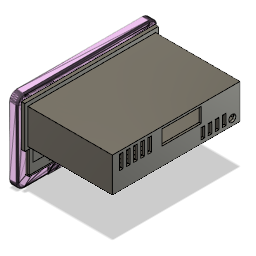
Headunit (Autodesk Fusion 360 design; units mm, degrees)
Autodesk Fusion 360 part; units mm, degrees
sketch "Sketch1" plane through (0, 0, 0) normal (0, 1, 0) x (1, 0, 0)
  line L0 (50, 100) -> (50, -80)
  line L1 (50, -80) -> (1, -80)
  line L2 (1, -80) -> (1, 100)
  line L3 (1, 100) -> (50, 100)
  constraint vertical L0
  constraint perpendicular L0 L1
  constraint perpendicular L1 L2
  constraint perpendicular L0 L3
extrude "Extrude1" add sketch "Sketch1" along normal blind 120 makes body 1
move_body "Move1" bodies 1 to x (0, 1, 0) y (-1, 0, 0) z (0, 0, 1) at (1, -1, 0)
shell "Shell1" thickness 3 removed faces 1 at (-119, 16.3333, -40) on bodies 1
hole "Hole1" at (1, 9.462, -88.8888) direction (-1, 0, 0) diameter 10 depth 60 tip angle 118 bodies 1
sketch "Sketch2" plane through (1, 0, 0) normal (1, 0, 0) x (0, 0, -1)
  circle A0 centre (88.8888, 9.462) radius 5
  line L0 (-80, 0) -> (100, 0)
  line L1 (100, 0) -> (100, 49)
  line L2 (100, 49) -> (-80, 49)
  line L3 (-80, 49) -> (-80, 0)
  line L4 (-60, 40) -> (-55.5469, 40)
  line L5 (-55.5469, 40) -> (-55.5469, 10)
  line L6 (-55.5469, 10) -> (-60, 10)
  line L7 (-60, 10) -> (-60, 40)
  constraint perpendicular L3 L4
  constraint perpendicular L4 L5
  constraint perpendicular L5 L6
  constraint perpendicular L4 L7
extrude "Extrude2" add sketch "Sketch2" along normal blind 40 contours L4 L5 L6 L7 bodies 1
delete_face "DeleteFace1" 1 faces at (14.3333, 20, 60) on bodies 1
sketch "Sketch5" plane through (1, 0, 0) normal (1, 0, 0) x (0, 0, -1)
  circle A0 centre (88.8888, 9.462) radius 5
  line L0 (-80, 49) -> (-80, 0)
  line L1 (-80, 0) -> (100, 0)
  line L2 (100, 0) -> (100, 49)
  line L3 (100, 49) -> (-80, 49)
  line L4 (-70, 40) -> (-64.9792, 40)
  line L5 (-64.9792, 40) -> (-64.9792, 10)
  line L6 (-64.9792, 10) -> (-67.4896, 10)
  line L7 (-67.4896, 10) -> (-70, 10)
  line L8 (-70, 10) -> (-70, 40)
  line L9 (-60, 40) -> (-54.6378, 40)
  line L10 (-54.6378, 40) -> (-54.6378, 10)
  line L11 (-54.6378, 10) -> (-60, 10)
  line L12 (-60, 10) -> (-60, 40)
  line L13 (-50, 40) -> (-44.6795, 40)
  line L14 (-44.6795, 40) -> (-44.6795, 10)
  line L15 (-44.6795, 10) -> (-47.3397, 10)
  line L16 (-47.3397, 10) -> (-50, 10)
  line L17 (-50, 10) -> (-50, 40)
  line L18 (-40, 40) -> (-34.7211, 40)
  line L19 (-34.7211, 40) -> (-34.7211, 10)
  line L20 (-34.7211, 10) -> (-40, 10)
  line L21 (-40, 10) -> (-40, 40)
  line L22 (-30, 40) -> (-24.7628, 40)
  line L23 (-24.7628, 40) -> (-24.7628, 10)
  line L24 (-24.7628, 10) -> (-30, 10)
  line L25 (-30, 10) -> (-30, 40)
  line L26 (-20, 40) -> (-14.8044, 40)
  line L27 (-14.8044, 40) -> (-14.8044, 10)
  line L28 (-14.8044, 10) -> (-20, 10)
  line L29 (-20, 10) -> (-20, 40)
  constraint parallel L3 L4
  constraint perpendicular L4 L5
  constraint perpendicular L5 L6
  constraint perpendicular L4 L8
  constraint perpendicular L5 L9
  constraint perpendicular L9 L10
  constraint perpendicular L10 L11
  constraint perpendicular L9 L12
  constraint perpendicular L10 L13
  constraint perpendicular L13 L14
  constraint perpendicular L14 L15
  constraint perpendicular L14 L16
  constraint perpendicular L13 L17
  constraint perpendicular L14 L18
  constraint perpendicular L18 L19
  constraint perpendicular L19 L20
  constraint perpendicular L18 L21
  constraint perpendicular L19 L22
  constraint perpendicular L22 L23
  constraint perpendicular L19 L24
  constraint perpendicular L22 L25
  constraint perpendicular L23 L26
  constraint perpendicular L26 L27
  constraint perpendicular L27 L28
  constraint perpendicular L26 L29
extrude "Extrude4" cut sketch "Sketch5" against normal blind 30 contours L4 L5 L6 L7 L8 | L9 L10 L11 L12 | L13 L14 L15 L16 L17 | L18 L19 L20 L21 | L22 L23 L24 L25 | L26 L27 L28 L29 bodies 1
sketch "Sketch6" plane through (-119, 0, 0) normal (-1, 0, 0) x (0, 0, 1)
  line L0 (-97, 3) -> (-97, 46)
  line L1 (-97, 46) -> (77, 46)
  line L2 (77, 46) -> (77, 3)
  line L3 (77, 3) -> (-97, 3)
  line L4 (-100, 0) -> (80, 0)
  line L5 (80, 0) -> (80, 49)
  line L6 (80, 49) -> (-100, 49)
  line L7 (-100, 49) -> (-100, 0)
  line L8 (-104.1759, 54.472) -> (84.2667, 54.472)
  line L9 (84.2667, 54.472) -> (84.2667, -4.1291)
  line L10 (84.2667, -4.1291) -> (-103.7929, -4.1291)
  line L11 (-103.7929, -4.1291) -> (-104.1759, 54.472)
  constraint parallel L6 L8
  constraint perpendicular L8 L9
  constraint perpendicular L9 L10
extrude "Extrude5" add sketch "Sketch6" along normal blind 5 separate body contours L8 L9 L10 L11 makes body 2
move_body "Move4" bodies 2 to x (1, 0, 0) y (0, 1, 0) z (0, 0, 1) at (1, 0, 0)
mesh "Mesh1" [no effect]
sketch "Sketch7" plane through (-2, 0, 0) normal (-1, 0, 0) x (0, 0, 1)
  line L0 (44.6795, 10) -> (44.6795, 40)
  line L1 (44.6795, 40) -> (50, 40)
  line L2 (50, 40) -> (50, 10)
  line L3 (50, 10) -> (44.6795, 10)
  line L4 (14.8044, 10) -> (14.8044, 40)
  line L5 (14.8044, 40) -> (20, 40)
  line L6 (20, 40) -> (20, 10)
  line L7 (20, 10) -> (14.8044, 10)
  line L8 (54.6378, 10) -> (54.6378, 40)
  line L9 (54.6378, 40) -> (60, 40)
  line L10 (60, 40) -> (60, 10)
  line L11 (60, 10) -> (54.6378, 10)
  line L12 (34.7211, 10) -> (34.7211, 40)
  line L13 (34.7211, 40) -> (40, 40)
  line L14 (40, 40) -> (40, 10)
  line L15 (40, 10) -> (34.7211, 10)
  line L16 (24.7628, 10) -> (24.7628, 40)
  line L17 (24.7628, 40) -> (30, 40)
  line L18 (30, 40) -> (30, 10)
  line L19 (30, 10) -> (24.7628, 10)
  line L20 (64.9792, 10) -> (64.9792, 40)
  line L21 (64.9792, 40) -> (70, 40)
  line L22 (70, 40) -> (70, 10)
  line L23 (70, 10) -> (64.9792, 10)
  circle A0 centre (-88.8888, 9.462) radius 5
  line L24 (-97, 3) -> (77, 3)
  line L25 (77, 3) -> (77, 46)
  line L26 (77, 46) -> (-97, 46)
  line L27 (-97, 46) -> (-97, 3)
  line L28 (-97, 24.9908) -> (-92, 24.9908)
  line L29 (-92, 24.9908) -> (-92, 28)
  line L30 (-97, 28) -> (-97, 24.9908)
  line L31 (-97, 24.9908) -> (-97, 23.492)
  line L32 (-97, 24.9908) -> (-97, 22.5)
  line L33 (-92, 22.5) -> (-97, 22.5)
  line L34 (-92, 22.5) -> (-92, 20.5)
  line L35 (-92, 20.5) -> (-91.9643, 13.4043)
  line L36 (-91.9643, 13.4043) -> (-97, 13.4)
  line L37 (-97, 22.5) -> (-97, 13.4)
  line L38 (-92, 28) -> (-92, 46)
  line L39 (-97, 46) -> (-97, 24.9908)
  constraint coincident L27 L28.start
  constraint perpendicular L27 L28
  constraint perpendicular L28 L29
  constraint coincident L27 L30.start
  constraint coincident L27 L31.end
  constraint coincident L27 L32.end
  constraint perpendicular L27 L33
  constraint coincident A0 L35.end
  constraint coincident L27 L36.end
  constraint coincident L26 L38.end
  constraint coincident L26.end L27.start
extrude "Extrude6" add sketch "Sketch7" along normal blind 100 contours L27 L33 L34 L35 L36 L37 | L26 L27 L28 L29 L30 L38 L39 bodies 1
sketch "Sketch8" plane through (-2, 0, 0) normal (-1, 0, 0) x (0, 0, 1)
  line L0 (-91.9643, 13.4043) -> (-97, 13.4)
  line L1 (-97, 13.4) -> (-97, 3)
  line L2 (-97, 3) -> (77, 3)
  line L3 (77, 3) -> (77, 46)
  line L4 (77, 46) -> (-92, 46)
  line L5 (-92, 46) -> (-92, 24.9908)
  line L6 (-92, 24.9908) -> (-97, 24.9908)
  line L7 (-97, 24.9908) -> (-97, 22.5)
  line L8 (-97, 22.5) -> (-92, 22.5)
  line L9 (-92, 22.5) -> (-92, 20.5)
  line L10 (-92, 20.5) -> (-91.9643, 13.4043)
  circle A0 centre (-88.8888, 9.462) radius 5
  line L11 (64.9792, 10) -> (64.9792, 40)
  line L12 (64.9792, 40) -> (70, 40)
  line L13 (70, 40) -> (70, 10)
  line L14 (70, 10) -> (64.9792, 10)
  line L15 (24.7628, 10) -> (24.7628, 40)
  line L16 (24.7628, 40) -> (30, 40)
  line L17 (30, 40) -> (30, 10)
  line L18 (30, 10) -> (24.7628, 10)
  line L19 (34.7211, 10) -> (34.7211, 40)
  line L20 (34.7211, 40) -> (40, 40)
  line L21 (40, 40) -> (40, 10)
  line L22 (40, 10) -> (34.7211, 10)
  line L23 (54.6378, 10) -> (54.6378, 40)
  line L24 (54.6378, 40) -> (60, 40)
  line L25 (60, 40) -> (60, 10)
  line L26 (60, 10) -> (54.6378, 10)
  line L27 (14.8044, 10) -> (14.8044, 40)
  line L28 (14.8044, 40) -> (20, 40)
  line L29 (20, 40) -> (20, 10)
  line L30 (20, 10) -> (14.8044, 10)
  line L31 (44.6795, 10) -> (44.6795, 40)
  line L32 (44.6795, 40) -> (50, 40)
  line L33 (50, 40) -> (50, 10)
  line L34 (50, 10) -> (44.6795, 10)
  line L35 (77, 25.0463) -> (71.9692, 24.9908)
  line L36 (71.9692, 24.9908) -> (71.9692, 46)
  line L37 (77, 22.1504) -> (72, 22.1504)
  line L38 (72, 22.1504) -> (72, 3)
  constraint coincident L3 L35.start
  constraint coincident L4 L36.end
  constraint perpendicular L4 L36
  constraint coincident L3 L37.start
  constraint perpendicular L3 L37
  constraint coincident L2 L38.end
extrude "Extrude7" add sketch "Sketch8" along normal blind 100 contours L3 L4 L35 L36 bodies 1
sketch "Sketch9" plane through (-2, 0, 0) normal (-1, 0, 0) x (0, 0, 1)
  line L0 (71.9692, 24.9908) -> (71.9692, 46)
  line L1 (71.9692, 46) -> (-92, 46)
  line L2 (-92, 46) -> (-92, 24.9908)
  line L3 (-92, 24.9908) -> (-97, 24.9908)
  line L4 (-97, 24.9908) -> (-97, 22.5)
  line L5 (-97, 22.5) -> (-92, 22.5)
  line L6 (-92, 22.5) -> (-92, 20.5)
  line L7 (-92, 20.5) -> (-91.9643, 13.4043)
  circle A0 centre (-88.8888, 9.462) radius 5
  line L8 (-91.9643, 13.4043) -> (-97, 13.4)
  line L9 (-97, 13.4) -> (-97, 3)
  line L10 (-97, 3) -> (77, 3)
  line L11 (77, 3) -> (77, 25.0463)
  line L12 (77, 25.0463) -> (71.9692, 24.9908)
  line L13 (64.9792, 10) -> (64.9792, 40)
  line L14 (64.9792, 40) -> (70, 40)
  line L15 (70, 40) -> (70, 10)
  line L16 (70, 10) -> (64.9792, 10)
  line L17 (24.7628, 10) -> (24.7628, 40)
  line L18 (24.7628, 40) -> (30, 40)
  line L19 (30, 40) -> (30, 10)
  line L20 (30, 10) -> (24.7628, 10)
  line L21 (34.7211, 10) -> (34.7211, 40)
  line L22 (34.7211, 40) -> (40, 40)
  line L23 (40, 40) -> (40, 10)
  line L24 (40, 10) -> (34.7211, 10)
  line L25 (54.6378, 10) -> (54.6378, 40)
  line L26 (54.6378, 40) -> (60, 40)
  line L27 (60, 40) -> (60, 10)
  line L28 (60, 10) -> (54.6378, 10)
  line L29 (14.8044, 10) -> (14.8044, 40)
  line L30 (14.8044, 40) -> (20, 40)
  line L31 (20, 40) -> (20, 10)
  line L32 (20, 10) -> (14.8044, 10)
  line L33 (44.6795, 10) -> (44.6795, 40)
  line L34 (44.6795, 40) -> (50, 40)
  line L35 (50, 40) -> (50, 10)
  line L36 (50, 10) -> (44.6795, 10)
  line L37 (77, 22.5204) -> (72, 22.5204)
  line L38 (72, 22.5204) -> (72, 3)
  constraint coincident L11 L37.start
  constraint perpendicular L11 L37
  constraint coincident L10 L38.end
extrude "Extrude8" add sketch "Sketch9" along normal blind 100 contours L10 L11 L37 L38 bodies 1
sketch "Sketch10" plane through (-2, 0, 0) normal (-1, 0, 0) x (0, 0, 1)
  line L0 (44.6795, 10) -> (44.6795, 40)
  line L1 (44.6795, 40) -> (50, 40)
  line L2 (50, 40) -> (50, 10)
  line L3 (50, 10) -> (44.6795, 10)
  line L4 (14.8044, 10) -> (14.8044, 40)
  line L5 (14.8044, 40) -> (20, 40)
  line L6 (20, 40) -> (20, 10)
  line L7 (20, 10) -> (14.8044, 10)
  line L8 (54.6378, 10) -> (54.6378, 40)
  line L9 (54.6378, 40) -> (60, 40)
  line L10 (60, 40) -> (60, 10)
  line L11 (60, 10) -> (54.6378, 10)
  line L12 (34.7211, 10) -> (34.7211, 40)
  line L13 (34.7211, 40) -> (40, 40)
  line L14 (40, 40) -> (40, 10)
  line L15 (40, 10) -> (34.7211, 10)
  line L16 (24.7628, 10) -> (24.7628, 40)
  line L17 (24.7628, 40) -> (30, 40)
  line L18 (30, 40) -> (30, 10)
  line L19 (30, 10) -> (24.7628, 10)
  line L20 (64.9792, 10) -> (64.9792, 40)
  line L21 (64.9792, 40) -> (70, 40)
  line L22 (70, 40) -> (70, 10)
  line L23 (70, 10) -> (64.9792, 10)
  line L24 (72, 3) -> (72, 22.5204)
  line L25 (72, 22.5204) -> (77, 22.5204)
  line L26 (77, 22.5204) -> (77, 25.0463)
  line L27 (77, 25.0463) -> (71.9692, 24.9908)
  line L28 (71.9692, 24.9908) -> (71.9692, 46)
  line L29 (71.9692, 46) -> (-92, 46)
  line L30 (-92, 46) -> (-92, 24.9908)
  line L31 (-92, 24.9908) -> (-97, 24.9908)
  line L32 (-97, 24.9908) -> (-97, 22.5)
  line L33 (-97, 22.5) -> (-92, 22.5)
  line L34 (-92, 22.5) -> (-92, 20.5)
  line L35 (-92, 20.5) -> (-91.9643, 13.4043)
  circle A0 centre (-88.8888, 9.462) radius 5
  line L36 (-91.9643, 13.4043) -> (-97, 13.4)
  line L37 (-97, 13.4) -> (-97, 3)
  line L38 (-97, 3) -> (72, 3)
  line L39 (-97, 24.9908) -> (77, 25.0463)
  line L40 (77, 22.5204) -> (-97, 22.5)
  line L41 (-97, 24.9908) -> (-97, 22.5)
  line L42 (-97, 24.9908) -> (77, 25.0463)
  line L43 (77, 25.0463) -> (-97, 24.9908)
  line L44 (-97, 22.5) -> (77, 22.5204)
  constraint coincident L31.end L32.start
  constraint coincident L26.end L27.start
  constraint coincident L25.end L26.start
  constraint coincident L32.end L33.start
extrude "Extrude9" add sketch "Sketch10" along normal blind 100 separate body contours L0 L14 L39 L40 L42 L43 L44 | L0 L2 L39 L40 L42 L43 L44 | L2 L8 L39 L40 L42 L43 L44 | L12 L14 L39 L40 L42 L43 L44 | L8 L10 L39 L40 L42 L43 L44 | L12 L18 L39 L40 L42 L43 L44 | L10 L20 L39 L40 L42 L43 L44 | L16 L18 L39 L40 L42 L43 L44 | L20 L22 L39 L40 L42 L43 L44 | L6 L16 L39 L40 L42 L43 L44 | L22 L25 L26 L27 L28 L39 L40 L42 L43 L44 | L4 L6 L39 L40 L42 L43 L44 | L4 L31 L32 L33 L39 L40 L41 L42 L43 L44 makes body 3
sketch "Sketch11" plane through (-102, 0, 0) normal (-1, 0, 0) x (0, 0, 1)
  line L0 (-97, 22.5) -> (72, 22.5198)
  line L1 (72, 22.5198) -> (72, 22.5204)
  line L2 (72, 22.5204) -> (77, 22.5204)
  line L3 (77, 22.5204) -> (77, 25.0463)
  line L4 (77, 25.0463) -> (71.9692, 24.9908)
  line L5 (71.9692, 24.9908) -> (71.9692, 25.0447)
  line L6 (71.9692, 25.0447) -> (-92, 24.9924)
  line L7 (-92, 24.9924) -> (-92, 24.9908)
  line L8 (-92, 24.9908) -> (-97, 24.9908)
  line L9 (-97, 24.9908) -> (-97, 22.5)
  line L10 (-92, 46) -> (71.9692, 46)
  line L11 (-45.0737, 28) -> (-45.0727, 25.0074)
  line L12 (-45.0727, 25.0074) -> (-45.0727, 46)
  line L13 (-45.0727, 25.0074) -> (10.0774, 25.0249)
  line L14 (10.0774, 46) -> (-45.0727, 46)
  line L15 (-45.0727, 25.0074) -> (10.0774, 25.0249)
  line L16 (10.0774, 46) -> (-45.0727, 46)
  line L17 (-45.0737, 28) -> (-45.0727, 25.0074)
  line L18 (10.0774, 25.0249) -> (10.0774, 46)
  constraint coincident L6 L11.end
  constraint perpendicular L6 L11
  constraint coincident L10 L12.end
  constraint perpendicular L10 L12
  constraint coincident L6 L13.end
  constraint parallel L6 L13
  constraint coincident L10 L14.start
  constraint parallel L13 L15
  constraint vertical L18
extrude "Extrude10" cut sketch "Sketch11" against normal blind 115 contours L6 L10 L11 L12 L13 L14 L15 L16 L17 L18 bodies 1
sketch "Sketch12" plane through (-2, 0, 0) normal (-1, 0, 0) x (0, 0, 1)
  line L0 (-45.0727, 25.0074) -> (-45.0727, 46)
  line L1 (-45.0727, 46) -> (-92, 46)
  line L2 (-92, 46) -> (-92, 24.9908)
  line L3 (-92, 24.9908) -> (-97, 24.9908)
  line L4 (-97, 24.9908) -> (-97, 22.5)
  line L5 (-97, 22.5) -> (-92, 22.5)
  line L6 (-92, 22.5) -> (-92, 20.5)
  line L7 (-92, 20.5) -> (-91.9643, 13.4043)
  circle A0 centre (-88.8888, 9.462) radius 5
  line L8 (-91.9643, 13.4043) -> (-97, 13.4)
  line L9 (-97, 13.4) -> (-97, 3)
  line L10 (-97, 3) -> (72, 3)
  line L11 (72, 3) -> (72, 22.5204)
  line L12 (72, 22.5204) -> (77, 22.5204)
  line L13 (77, 22.5204) -> (77, 25.0463)
  line L14 (77, 25.0463) -> (71.9692, 24.9908)
  line L15 (71.9692, 24.9908) -> (71.9692, 46)
  line L16 (71.9692, 46) -> (10.0774, 46)
  line L17 (10.0774, 46) -> (10.0774, 25.0249)
  line L18 (10.0774, 25.0249) -> (-45.0727, 25.0074)
  line L19 (44.6795, 10) -> (44.6795, 40)
  line L20 (44.6795, 40) -> (50, 40)
  line L21 (50, 40) -> (50, 10)
  line L22 (50, 10) -> (44.6795, 10)
  line L23 (14.8044, 10) -> (14.8044, 40)
  line L24 (14.8044, 40) -> (20, 40)
  line L25 (20, 40) -> (20, 10)
  line L26 (20, 10) -> (14.8044, 10)
  line L27 (54.6378, 10) -> (54.6378, 40)
  line L28 (54.6378, 40) -> (60, 40)
  line L29 (60, 40) -> (60, 10)
  line L30 (60, 10) -> (54.6378, 10)
  line L31 (34.7211, 10) -> (34.7211, 40)
  line L32 (34.7211, 40) -> (40, 40)
  line L33 (40, 40) -> (40, 10)
  line L34 (40, 10) -> (34.7211, 10)
  line L35 (24.7628, 10) -> (24.7628, 40)
  line L36 (24.7628, 40) -> (30, 40)
  line L37 (30, 40) -> (30, 10)
  line L38 (30, 10) -> (24.7628, 10)
  line L39 (64.9792, 10) -> (64.9792, 40)
  line L40 (64.9792, 40) -> (70, 40)
  line L41 (70, 40) -> (70, 10)
  line L42 (70, 10) -> (64.9792, 10)
  line L43 (-91.9643, 13.4043) -> (-92, 20.5)
  line L44 (-92, 22.5) -> (-92, 20.5)
  line L45 (-91.9643, 13.4043) -> (-92, 20.5)
  constraint coincident L7.end L8.start
  constraint coincident L6.end L7.start
  constraint coincident L5.end L6.start
extrude "Extrude11" add sketch "Sketch12" against normal blind 3 contours L19 L20 L21 L22 | L23 L24 L25 L26 | L27 L28 L29 L30 | L31 L32 L33 L34 | L35 L36 L37 L38 | L39 L40 L41 L42 bodies 1
sketch "Sketch13" plane through (1, 0, 0) normal (1, 0, 0) x (0, 0, -1)
  line L0 (-10.0774, 25.0249) -> (-10.0774, 46)
  line L1 (-10.0774, 46) -> (45.0727, 46)
  line L2 (45.0727, 46) -> (45.0727, 25.0074)
  line L3 (45.0727, 25.0074) -> (-10.0774, 25.0249)
  circle A0 centre (88.8888, 9.462) radius 5
  line L4 (-80, 49) -> (-80, 0)
  line L5 (-80, 0) -> (100, 0)
  line L6 (100, 0) -> (100, 49)
  line L7 (100, 49) -> (-80, 49)
  line L8 (-70, 45) -> (-65, 45)
  line L9 (-65, 45) -> (-65, 25)
  line L10 (-65, 25) -> (-70, 25)
  line L11 (-70, 25) -> (-70, 45)
  line L12 (-60, 45) -> (-55, 45)
  line L13 (-55, 45) -> (-55, 25)
  line L14 (-55, 25) -> (-60, 25)
  line L15 (-60, 25) -> (-60, 45)
  line L16 (-50, 45) -> (-45, 45)
  line L17 (-45, 45) -> (-45, 25)
  line L18 (-45, 25) -> (-50, 25)
  line L19 (-50, 25) -> (-50, 45)
  line L20 (-40, 45) -> (-35, 45)
  line L21 (-35, 45) -> (-35, 25)
  line L22 (-35, 25) -> (-40, 25)
  line L23 (-40, 25) -> (-40, 45)
  line L24 (-30, 45) -> (-25, 45)
  line L25 (-25, 45) -> (-25, 25)
  line L26 (-25, 25) -> (-30, 25)
  line L27 (-30, 25) -> (-30, 45)
  constraint horizontal L8
  constraint vertical L9
  constraint horizontal L10
  constraint vertical L11
  constraint horizontal L12
  constraint vertical L13
  constraint horizontal L14
  constraint vertical L15
  constraint horizontal L16
  constraint vertical L17
  constraint horizontal L18
  constraint vertical L19
  constraint horizontal L20
  constraint vertical L21
  constraint horizontal L22
  constraint vertical L23
  constraint horizontal L24
  constraint vertical L25
  constraint horizontal L26
  constraint vertical L27
extrude "Extrude12" cut sketch "Sketch13" against normal blind 7 contours L8 L9 L10 L11 | L12 L13 L14 L15 | L16 L17 L18 L19 | L20 L21 L22 L23 | L24 L25 L26 L27 bodies 1
sketch "Sketch14" plane through (-2, 0, 0) normal (-1, 0, 0) x (0, 0, 1)
  line L0 (45, 25) -> (45, 45)
  line L1 (45, 45) -> (50, 45)
  line L2 (50, 45) -> (50, 25)
  line L3 (50, 25) -> (45, 25)
  line L4 (25, 25) -> (25, 45)
  line L5 (25, 45) -> (30, 45)
  line L6 (30, 45) -> (30, 25)
  line L7 (30, 25) -> (25, 25)
  line L8 (55, 25) -> (55, 45)
  line L9 (55, 45) -> (60, 45)
  line L10 (60, 45) -> (60, 25)
  line L11 (60, 25) -> (55, 25)
  line L12 (35, 25) -> (35, 45)
  line L13 (35, 45) -> (40, 45)
  line L14 (40, 45) -> (40, 25)
  line L15 (40, 25) -> (35, 25)
  line L16 (65, 25) -> (65, 45)
  line L17 (65, 45) -> (70, 45)
  line L18 (70, 45) -> (70, 25)
  line L19 (70, 25) -> (65, 25)
  line L20 (-45.0727, 25.0074) -> (-45.0727, 46)
  line L21 (-45.0727, 46) -> (-92, 46)
  line L22 (-92, 46) -> (-92, 24.9908)
  line L23 (-92, 24.9908) -> (-97, 24.9908)
  line L24 (-97, 24.9908) -> (-97, 22.5)
  line L25 (-97, 22.5) -> (-92, 22.5)
  line L26 (-92, 22.5) -> (-92, 20.5)
  line L27 (-92, 20.5) -> (-91.9643, 13.4043)
  circle A0 centre (-88.8888, 9.462) radius 5
  line L28 (-91.9643, 13.4043) -> (-97, 13.4)
  line L29 (-97, 13.4) -> (-97, 3)
  line L30 (-97, 3) -> (72, 3)
  line L31 (72, 3) -> (72, 22.5204)
  line L32 (72, 22.5204) -> (77, 22.5204)
  line L33 (77, 22.5204) -> (77, 25.0463)
  line L34 (77, 25.0463) -> (71.9692, 24.9908)
  line L35 (71.9692, 24.9908) -> (71.9692, 46)
  line L36 (71.9692, 46) -> (10.0774, 46)
  line L37 (10.0774, 46) -> (10.0774, 25.0249)
  line L38 (10.0774, 25.0249) -> (-45.0727, 25.0074)
  line L39 (-97, 22.5) -> (72, 22.5198)
  line L40 (-47.8629, 22.5058) -> (-45.2341, 22.5061)
  line L41 (-40.1585, 22.5099) -> (-35.1082, 22.5099)
  line L42 (-35.1082, 22.5099) -> (-35.1082, 3)
  line L43 (-35.1082, 3) -> (-40.1585, 3)
  line L44 (-40.1585, 3) -> (-40.1585, 22.5099)
  constraint coincident L39 L40.end
  constraint coincident L39 L40.start
  constraint horizontal L41
  constraint vertical L42
  constraint horizontal L43
  constraint vertical L44
  constraint coincident L30 L42.end
extrude "Extrude13" add sketch "Sketch14" along normal blind 100 contours L30 L39 L42 L43 L44 bodies 1
sketch "Sketch15" plane through (0, 25.0217, -0.008) normal (0, 1, -0.000319) x (-1, 0, 0)
  line L0 (2, 71.9771) -> (2, -91.992)
  line L1 (2, -91.992) -> (102, -91.992)
  line L2 (102, -91.992) -> (102, 71.9771)
  line L3 (102, 71.9771) -> (2, 71.9771)
  line L4 (50, -25) -> (52, -25)
  line L5 (140, -35) -> (144, -35)
  line L6 (144, -35) -> (144, -60)
  line L7 (144, -60) -> (165.6691, -72.7647)
  line L8 (165.6691, -72.7647) -> (163.6374, -76.2137)
  line L9 (163.6374, -76.2137) -> (142, -63.4677)
  line L10 (142, -63.4677) -> (120.1739, -75.6587)
  line L11 (120.1739, -75.6587) -> (118.1983, -72.1217)
  line L12 (118.1983, -72.1217) -> (140.0281, -59.9286)
  line L13 (140.0281, -59.9286) -> (140, -35)
  constraint perpendicular L2 L4
  constraint horizontal L5
  constraint perpendicular L5 L6
  constraint perpendicular L7 L8
  constraint perpendicular L8 L9
  constraint perpendicular L10 L11
  constraint perpendicular L11 L12
extrude "Extrude14" add sketch "Sketch15" along normal blind 2 separate body contours L5 L6 L7 L8 L9 L10 L11 L12 L13 makes body 4
hole "Hole2" at (-46.8993, 25.0008, -65.6257) direction (0, -1, 0.000319) diameter 50 depth 40 tip angle 118 bodies 3
move_body "Move5" bodies 4 to x (1, 0, 0) y (0, 1, 0) z (0, 0, 1) at (95.236, -2.8131, -4.7896)
sketch "Sketch16" plane through (-123, 0, 0) normal (-1, 0, 0) x (0, 0, 1)
  line L0 (-100, 0) -> (-100, 49)
  line L1 (-100, 49) -> (80, 49)
  line L2 (80, 0) -> (-100, 0)
  line L3 (-103.7929, -4.1291) -> (84.2667, -4.1291)
  line L4 (84.2667, -4.1291) -> (84.2667, 54.472)
  line L5 (84.2667, 54.472) -> (-104.1759, 54.472)
  line L6 (-104.1759, 54.472) -> (-103.7929, -4.1291)
  point P0 (-97, 46)
  point P1 (-97, 3)
  point P2 (77, 46)
  point P3 (77, 3)
sketch "Sketch17" plane through (-102, 0, 0) normal (-1, 0, 0) x (0, 0, 1)
  line L0 (-97, 22.5) -> (72, 22.5198)
  line L1 (72, 22.5198) -> (72, 22.5204)
  line L2 (72, 22.5204) -> (77, 22.5204)
  line L3 (77, 22.5204) -> (77, 25.0463)
  line L4 (77, 25.0463) -> (71.9692, 24.9908)
  line L5 (71.9692, 24.9908) -> (71.9692, 25.0447)
  line L6 (71.9692, 25.0447) -> (-92, 24.9924)
  line L7 (-92, 24.9924) -> (-92, 24.9908)
  line L8 (-92, 24.9908) -> (-97, 24.9908)
  line L9 (-97, 24.9908) -> (-97, 22.5)
  line L10 (-97, 46) -> (77, 46)
  line L11 (77, 46) -> (77, 3)
  line L12 (77, 3) -> (-97, 3)
  line L13 (-97, 3) -> (-97, 46)
  point P0 (-97, 46)
  point P1 (77, 46)
  point P2 (77, 3)
  point P3 (-97, 3)
  constraint coincident P0 L10.start
  constraint coincident P1 L10.end
  constraint coincident P2 L11.end
  constraint coincident P3 L12.end
extrude "Extrude15" add sketch "Sketch17" along normal blind 17 bodies 3
extrude "Extrude16" add 1 faces at (-38.1728, 24.1878, -69.9708) along direction (0, 1, -0.000319) blind 1 on bodies 4 bodies 4 3
sketch "Sketch18" plane through (-2, 0, 0) normal (-1, 0, 0) x (0, 0, 1)
  line L0 (-35.1082, 22.5072) -> (-35.1082, 3)
  line L1 (-35.1082, 3) -> (72, 3)
  line L2 (72, 3) -> (72, 22.5204)
  line L3 (72, 22.5204) -> (77, 22.5204)
  line L4 (77, 22.5204) -> (77, 25.0463)
  line L5 (77, 25.0463) -> (71.9692, 24.9908)
  line L6 (71.9692, 24.9908) -> (71.9692, 46)
  line L7 (71.9692, 46) -> (10.0774, 46)
  line L8 (10.0774, 46) -> (10.0774, 25.0249)
  line L9 (10.0774, 25.0249) -> (-45.0727, 25.0074)
  line L10 (-45.0727, 25.0074) -> (-45.0727, 46)
  line L11 (-45.0727, 46) -> (-92, 46)
  line L12 (-92, 46) -> (-92, 24.9908)
  line L13 (-92, 24.9908) -> (-97, 24.9908)
  line L14 (-97, 24.9908) -> (-97, 22.5)
  line L15 (-97, 22.5) -> (-92, 22.5)
  line L16 (-92, 22.5) -> (-92, 20.5)
  line L17 (-92, 20.5) -> (-91.9643, 13.4043)
  circle A0 centre (-88.8888, 9.462) radius 5
  line L18 (-91.9643, 13.4043) -> (-97, 13.4)
  line L19 (-97, 13.4) -> (-97, 3)
  line L20 (-97, 3) -> (-40.1585, 3)
  line L21 (-40.1585, 3) -> (-40.1585, 22.5067)
  line L22 (-40.1585, 22.5067) -> (-35.1082, 22.5072)
  line L23 (45, 25) -> (45, 45)
  line L24 (45, 45) -> (50, 45)
  line L25 (50, 45) -> (50, 25)
  line L26 (50, 25) -> (45, 25)
  line L27 (25, 25) -> (25, 45)
  line L28 (25, 45) -> (30, 45)
  line L29 (30, 45) -> (30, 25)
  line L30 (30, 25) -> (25, 25)
  line L31 (55, 25) -> (55, 45)
  line L32 (55, 45) -> (60, 45)
  line L33 (60, 45) -> (60, 25)
  line L34 (60, 25) -> (55, 25)
  line L35 (35, 25) -> (35, 45)
  line L36 (35, 45) -> (40, 45)
  line L37 (40, 45) -> (40, 25)
  line L38 (40, 25) -> (35, 25)
  line L39 (65, 25) -> (65, 45)
  line L40 (65, 45) -> (70, 45)
  line L41 (70, 45) -> (70, 25)
  line L42 (70, 25) -> (65, 25)
  line L43 (-80, 20) -> (-75.0292, 20)
  line L44 (-75.0292, 20) -> (-75.0292, 4.9966)
  line L45 (-75.0292, 4.9966) -> (-80.0571, 4.9966)
  line L46 (-80.0571, 4.9966) -> (-80, 20)
  line L47 (-69.9982, 20) -> (-65, 20)
  line L48 (-65, 20) -> (-65, 4.9966)
  line L49 (-65, 4.9966) -> (-70.0698, 4.9966)
  line L50 (-70.0698, 4.9966) -> (-69.9982, 20)
  line L51 (-59.9752, 20) -> (-54.9994, 20)
  line L52 (-54.9994, 20) -> (-54.9994, 4.9966)
  line L53 (-54.9994, 4.9966) -> (-60.011, 4.9966)
  line L54 (-60.011, 4.9966) -> (-59.9752, 20)
  line L55 (-50, 20) -> (-45, 20)
  line L56 (-45, 20) -> (-45, 5)
  line L57 (-45, 5) -> (-50, 5)
  line L58 (-50, 5) -> (-50, 20)
  constraint parallel L20 L43
  constraint perpendicular L20 L44
  constraint perpendicular L44 L45
  constraint perpendicular L44 L47
  constraint perpendicular L47 L48
  constraint perpendicular L48 L49
  constraint perpendicular L51 L52
  constraint perpendicular L52 L53
  constraint perpendicular L21 L55
  constraint perpendicular L55 L56
  constraint perpendicular L56 L57
  constraint perpendicular L55 L58
extrude "Extrude17" cut sketch "Sketch18" against normal blind 5 contours L43 L44 L45 L46 | L47 L48 L49 L50 | L51 L52 L53 L54 | L55 L56 L57 L58 bodies 1
sketch "Sketch19" plane through (-119, 0, 0) normal (-1, 0, 0) x (0, 0, 1)
  line L0 (-97, 3) -> (77, 3)
  line L1 (77, 3) -> (77, 46)
  line L2 (77, 46) -> (-97, 46)
  line L3 (-97, 46) -> (-97, 3)
  line L4 (-97, 46) -> (-97, -39)
  line L5 (77, 46) -> (77, -39)
  line L6 (77, -39) -> (-97, -39)
  constraint coincident L2.end L3.start
  constraint perpendicular L2 L4
  constraint coincident L1.end L2.start
  constraint perpendicular L2 L5
  constraint perpendicular L4 L6
extrude "Extrude18" add sketch "Sketch19" along normal blind 3 bodies 4
sketch "Sketch20" plane through (-122, 0, 0) normal (-1, 0, 0) x (0, 0, 1)
  line L0 (77, 46) -> (-97, 46)
  line L1 (-97, 46) -> (-97, -39)
  line L2 (-97, -39) -> (77, -39)
  line L3 (77, -39) -> (77, 46)
  line L4 (-90, 40) -> (-90, 5)
  line L5 (-90, 5) -> (70, 5)
  line L6 (70, 5) -> (70, 40)
  line L7 (70, 40) -> (-90, 40)
  constraint perpendicular L0 L4
  constraint perpendicular L4 L5
  constraint perpendicular L5 L6
  constraint perpendicular L4 L7
extrude "Extrude19" cut sketch "Sketch20" against normal blind 20 contours L4 L5 L6 L7 bodies 4
extrude "Extrude20" add 1 faces at (-102, 24.1775, -20.1304) along direction (-1, 0, 0) blind 20 on bodies 4 bodies 4
extrude "Extrude21" add 2 faces at (-122, 24.1775, -20.1304) (-122, -24.3333, 16.6667) along direction (-1, 0, 0) blind 5 on bodies 4 bodies 4
sketch "Sketch21" plane through (-127, 0, 0) normal (-1, 0, 0) x (0, 0, 1)
  line L0 (70, 22.5196) -> (70, 5)
  line L1 (70, 5) -> (-90, 5)
  line L2 (-90, 5) -> (-90, 22.5008)
  line L3 (-90, 22.5008) -> (70, 22.5196)
  line L4 (70, 25.044) -> (-90, 24.9931)
  line L5 (-90, 24.9931) -> (-90, 40)
  line L6 (-90, 40) -> (70, 40)
  line L7 (70, 40) -> (70, 25.044)
  line L8 (77, 46) -> (-97, 46)
  line L9 (-97, 46) -> (-97, -39)
  line L10 (-97, -39) -> (77, -39)
  line L11 (77, -39) -> (77, 46)
  line L12 (-90, 5) -> (-90, -35)
  line L13 (-90, -35) -> (70, -35)
  line L14 (70, -35) -> (70, 5)
  constraint coincident L1.end L2.start
  constraint perpendicular L1 L12
  constraint perpendicular L12 L13
  constraint coincident L0.end L1.start
  constraint perpendicular L1 L14
extrude "Extrude22" cut sketch "Sketch21" against normal blind 5 contours L1 L12 L13 L14 bodies 4
sketch "Sketch23" plane through (-2, 0, 0) normal (-1, 0, 0) x (0, 0, 1)
  line L0 (-65, 20) -> (-65, 4.9966)
  line L1 (-65, 4.9966) -> (-70.0698, 4.9966)
  line L2 (-70.0698, 4.9966) -> (-69.9982, 20)
  line L3 (-69.9982, 20) -> (-65, 20)
  line L4 (-54.9994, 20) -> (-54.9994, 4.9966)
  line L5 (-54.9994, 4.9966) -> (-60.011, 4.9966)
  line L6 (-60.011, 4.9966) -> (-59.9752, 20)
  line L7 (-59.9752, 20) -> (-54.9994, 20)
  line L8 (-75.0292, 20) -> (-75.0292, 4.9966)
  line L9 (-75.0292, 4.9966) -> (-80.0571, 4.9966)
  line L10 (-80.0571, 4.9966) -> (-80, 20)
  line L11 (-80, 20) -> (-75.0292, 20)
  line L12 (-45, 20) -> (-45, 5)
  line L13 (-45, 5) -> (-50, 5)
  line L14 (-50, 5) -> (-50, 20)
  line L15 (-50, 20) -> (-45, 20)
  line L16 (-35.1082, 22.5072) -> (-35.1082, 3)
  line L17 (-35.1082, 3) -> (72, 3)
  line L18 (72, 3) -> (72, 22.5204)
  line L19 (72, 22.5204) -> (77, 22.5204)
  line L20 (77, 22.5204) -> (77, 25.0463)
  line L21 (77, 25.0463) -> (71.9692, 24.9908)
  line L22 (71.9692, 24.9908) -> (71.9692, 46)
  line L23 (71.9692, 46) -> (10.0774, 46)
  line L24 (10.0774, 46) -> (10.0774, 25.0249)
  line L25 (10.0774, 25.0249) -> (-45.0727, 25.0074)
  line L26 (-45.0727, 25.0074) -> (-45.0727, 46)
  line L27 (-45.0727, 46) -> (-92, 46)
  line L28 (-92, 46) -> (-92, 24.9908)
  line L29 (-92, 24.9908) -> (-97, 24.9908)
  line L30 (-97, 24.9908) -> (-97, 22.5)
  line L31 (-97, 22.5) -> (-92, 22.5)
  line L32 (-92, 22.5) -> (-92, 20.5)
  line L33 (-92, 20.5) -> (-91.9643, 13.4043)
  circle A0 centre (-88.8888, 9.462) radius 5
  line L34 (-91.9643, 13.4043) -> (-97, 13.4)
  line L35 (-97, 13.4) -> (-97, 3)
  line L36 (-97, 3) -> (-40.1585, 3)
  line L37 (-40.1585, 3) -> (-40.1585, 22.5067)
  line L38 (-40.1585, 22.5067) -> (-35.1082, 22.5072)
  line L39 (45, 25) -> (45, 45)
  line L40 (45, 45) -> (50, 45)
  line L41 (50, 45) -> (50, 25)
  line L42 (50, 25) -> (45, 25)
  line L43 (25, 25) -> (25, 45)
  line L44 (25, 45) -> (30, 45)
  line L45 (30, 45) -> (30, 25)
  line L46 (30, 25) -> (25, 25)
  line L47 (55, 25) -> (55, 45)
  line L48 (55, 45) -> (60, 45)
  line L49 (60, 45) -> (60, 25)
  line L50 (60, 25) -> (55, 25)
  line L51 (35, 25) -> (35, 45)
  line L52 (35, 45) -> (40, 45)
  line L53 (40, 45) -> (40, 25)
  line L54 (40, 25) -> (35, 25)
  line L55 (65, 25) -> (65, 45)
  line L56 (65, 45) -> (70, 45)
  line L57 (70, 45) -> (70, 25)
  line L58 (70, 25) -> (65, 25)
  line L59 (-97, 24.9908) -> (-97, 22.5)
  line L60 (77, 22.5204) -> (77, 25.0463)
  line L61 (77, 25.0463) -> (-97, 24.9908)
  line L62 (-97, 22.5) -> (-97, 24.9908)
  line L63 (-97, 22.5) -> (77, 22.5204)
  line L64 (77, 25.0463) -> (77, 22.5204)
  line L65 (-97, 24.9908) -> (-97, 22.5)
  constraint coincident L29.end L30.start
  constraint coincident L30.end L31.start
  constraint coincident L19.end L20.start
  constraint coincident L20.end L21.start
extrude "Extrude23" add sketch "Sketch23" along normal blind 110 separate body contours L19 L20 L21 L22 L25 L29 L30 L31 L38 L39 L41 L42 L43 L45 L46 L47 L49 L50 L51 L53 L54 L55 L57 L58 L59 L60 L61 L62 L63 L64 L65 makes body 5
sketch "Sketch24" plane through (-119, 0, 0) normal (-1, 0, 0) x (0, 0, 1)
  line L0 (-97, 3) -> (-97, 46)
  line L1 (-97, 46) -> (77, 46)
  line L2 (77, 46) -> (77, 3)
  line L3 (77, 3) -> (-97, 3)
  line L4 (-100, 0) -> (80, 0)
  line L5 (80, 0) -> (80, 49)
  line L6 (80, 49) -> (-100, 49)
  line L7 (-100, 49) -> (-100, 0)
  line L8 (-97, 46) -> (-97, 3)
  line L9 (77, 3) -> (77, 46)
  line L10 (-97, 46) -> (77, 46)
  line L11 (-97, 3) -> (77, 3)
  line L12 (-97, 46) -> (-97, 3)
  constraint coincident L0.end L1.start
  constraint coincident L0.start L3.end
  constraint coincident L2.end L3.start
  constraint coincident L1.end L2.start
extrude "Extrude24" add sketch "Sketch24" against normal blind 17 separate body contours L0 L1 L2 L3 L8 L9 L10 L11 L12 makes body 6
extrude "Extrude25" cut 1 faces at (-112, 24.1799, -23.3678) along direction (-1, 0, 0) blind 5 on bodies 5 bodies 6
move_face "OffsetFaces1" offset 5 1 faces at (-112, 23.3401, 1.6667) on bodies 6
hole "Hole3" at (-50.0587, 25.0005, -66.5207) direction (0, -1, 0.000319) diameter 50 depth 30 tip angle 118 bodies 5
extrude "Extrude26" add sketch "Sketch15" along normal blind 2 separate body contours L5 L6 L7 L8 L9 L10 L11 L12 L13 makes body 7
move_body "Move6" bodies 7 to x (1, 0, 0) y (0, 1, 0) z (0, 0, 1) at (92.4916, -2, -5.0045)
extrude "Extrude27" add 1 faces at (-40.9172, 25.001, -70.1857) along direction (0, -1, 0.000319) blind 0.5 on bodies 7 bodies 7 5
extrude "Extrude28" add 1 faces at (-119, 31.6667, -39) along direction (-1, 0, 0) blind 3 on bodies 6 bodies 6
sketch "Sketch25" plane through (0, 3, 0) normal (0, -1, 0) x (1, 0, 0)
  line L0 (-122, -97) -> (-102, -97)
  line L1 (-102, -97) -> (-102, 77)
  line L2 (-102, 77) -> (-122, 77)
  line L3 (-122, 77) -> (-122, -97)
  line L4 (-119, 77) -> (-122, 77)
  line L5 (-122, -97) -> (-119, -97)
  line L6 (-119, 77) -> (-119, -97)
  line L7 (-122, 77) -> (-122, -97)
  line L8 (-122, 77) -> (-119, 77)
  line L9 (-119, 77) -> (-119, -97)
  line L10 (-119, -97) -> (-122, -97)
  line L11 (-122, -97) -> (-122, 77)
  line L12 (-122, 77) -> (-119, 77)
  line L13 (-122, 77) -> (-122, -97)
  line L14 (-119, -97) -> (-122, -97)
  line L15 (-119, -97) -> (-119, 77)
  line L16 (-122, 77) -> (-119, 77)
  line L17 (-122, 77) -> (-122, -97)
  point P0 (-119, 77)
  point P1 (-119, -97)
  point P2 (-119, -97)
  constraint coincident P0 L4.start
  constraint coincident L2.end L3.start
  constraint coincident L0.start L3.end
  constraint coincident P2 P1
extrude "Extrude29" add sketch "Sketch25" along normal blind 40 contours L0 L2 L3 L4 L5 L6 L7 L8 L9 L10 L11 L12 L13 L14 L15 L16 L17 bodies 6
sketch "Sketch26" plane through (-122, 0, 0) normal (-1, 0, 0) x (0, 0, 1)
  line L0 (-97, 46) -> (-97, -37)
  line L1 (-97, -37) -> (77, -37)
  line L2 (77, -37) -> (77, 46)
  line L3 (77, 46) -> (-97, 46)
  line L4 (-91.4808, 41.6141) -> (71.8101, 41.6141)
  line L5 (71.8101, 41.6141) -> (71.8101, -33.0453)
  line L6 (71.8101, -33.0453) -> (-92.4703, -33.0453)
  line L7 (-92.4703, -33.0453) -> (-92.4703, 41.6141)
  line L8 (-92.4703, 41.6141) -> (-91.4808, 41.6141)
  constraint perpendicular L0 L4
  constraint perpendicular L4 L5
  constraint perpendicular L0 L6
  constraint perpendicular L4 L7
  constraint parallel L4 L8
extrude "Extrude30" cut sketch "Sketch26" against normal blind 30 contours L4 L5 L6 L7 L8 bodies 6
mesh "Mesh2" [no effect]
sketch "Sketch27" plane through (-122, 0, 0) normal (-1, 0, 0) x (0, 0, 1)
  line L0 (71.8101, -33.0453) -> (-92.4703, -33.0453)
  line L1 (-92.4703, -33.0453) -> (-92.4703, 41.6141)
  line L2 (-92.4703, 41.6141) -> (71.8101, 41.6141)
  line L3 (71.8101, 41.6141) -> (71.8101, -33.0453)
  line L4 (-97, 46) -> (-97, -37)
  line L5 (-97, -37) -> (77, -37)
  line L6 (77, -37) -> (77, 46)
  line L7 (77, 46) -> (-97, 46)
  line L8 (48.2535, 46) -> (48.2535, 30)
  line L9 (48.2535, 30) -> (71.8101, 30.5755)
  line L10 (48.7511, -33.0453) -> (48.7511, -24.1621)
  line L11 (48.7511, -24.1621) -> (71.8101, -23.9133)
  line L12 (-66.4467, -23.9133) -> (-66.1979, -33.0453)
  line L13 (-66.4467, -23.9133) -> (-90, -23.9133)
  line L14 (-66.4467, 30) -> (-66.6955, 46)
  line L15 (-66.4467, 30) -> (-90, 30)
  line L16 (-90, 30) -> (-97, 30)
  line L17 (-90, -23.9133) -> (-97, -23.9133)
  constraint coincident L7 L8.start
  constraint perpendicular L2 L8
  constraint coincident L3 L9.end
  constraint coincident L0 L10.start
  constraint perpendicular L0 L10
  constraint coincident L3 L11.end
  constraint coincident L0 L12.end
  constraint perpendicular L1 L13
  constraint coincident L7 L14.end
  constraint coincident L4 L16.end
  constraint perpendicular L1 L16
  constraint perpendicular L1 L17
extrude "Extrude31" add sketch "Sketch27" against normal blind 3 contours L0 L3 L10 L11 | L0 L1 L12 L13 L17 | L2 L3 L8 L9 | L1 L2 L14 L15 L16 bodies 6
